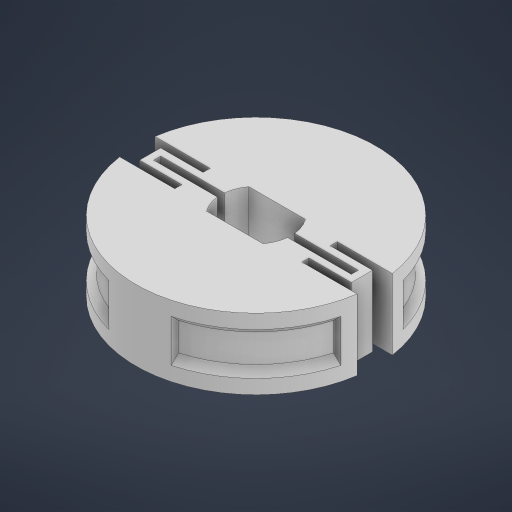
# Autodesk Inventor part: motor_grip
Saved by Autodesk Inventor 2024 (Build 280153000, 153)
## iProperties
Created: 2024-10-06
Part Number: motor_grip
Material: Generic
Document SubType Name: Modeling
Designer: loren
Density: 1 g/cm^3
Appearance: Default
Author: loren
## iProperties of the stored document shaft-grip_3DPrint.ipt
Created: 2026-02-06
Part Number: shaft-grip_3DPrint
Material: Generic
Document SubType Name: Modeling
Designer: lokies
Density: 1 g/cm^3
Appearance: Default
Author: lokies
Autodesk Inventor part; units mm, degrees
ref_plane "YZ Plane" through (0, 0, 0) normal (1, 0, 0) x (0, 1, 0)
ref_plane "XZ Plane" through (0, 0, 0) normal (0, 1, 0) x (-1, 0, 0)
ref_plane "XY Plane" through (0, 0, 0) normal (0, 0, 1) x (1, 0, 0)
sketch "Sketch1" plane through (0, 0, 0) normal (0, 0, 1) x (1, 0, 0)
  circle A0 centre (0, 0) radius 8.5
  circle A1 centre (0, 0) radius 2.5
  line L0 (-2, 1.5) -> (2, 1.5)
  line L1 (-2, -1.5) -> (2, -1.5)
  dimension "d0" = 17
  dimension "d42" = 5
  dimension "d43" = 3
  constraints: 4 end point, 4 point on circle, 2 centre point, 2 coincident, 2 horizontal, 1 parallel
  measures "d0" diameter of A0
  measures "d42" diameter of A1
  measures "d43" distance between parallel lines of L1 L0
extrude "Extrusion1" add sketch "Sketch1" along normal mid plane 5 contours A0 | L0 A1 | A1 L1
sketch "Sketch5" plane through (0, 0, 2.5) normal (0, 0, 1) x (1, 0, 0)
  line L0 (0, 0.25) -> (7, 0.25)
  line L1 (7, 0.25) -> (7, -0.25)
  line L2 (7, -0.25) -> (0, -0.25)
  line L3 (0, -0.25) -> (0, 0.25)
  circle A0 centre (0, 0) radius 8.5 projected
  line L4 (7.5, 0.75) -> (4.5, 0.75)
  line L5 (4.5, 0.75) -> (4.5, 1.25)
  line L6 (4.5, 1.25) -> (8.4076, 1.25)
  line L7 (7.5, -0.75) -> (4.5, -0.75)
  line L8 (4.5, -0.75) -> (4.5, -1.25)
  line L9 (4.5, -1.25) -> (8.4076, -1.25)
  line L10 (7.5, 0.75) -> (7.5, -0.75)
  point P0 (8.402, -1.287)
  point P1 (8.402, 1.287)
  dimension "d19" = 0.5
  dimension "d21" = 0.5
  dimension "d22" = 0.5
  dimension "d28" = 7
  dimension "d29" = 0.5
  dimension "d44" = 2.5
  dimension "d45" = 0.5
  constraints: 22 end point, 4 parallel, 3 horizontal, 3 perpendicular, 2 equal length, 2 point on circle, 1 coincident, 1 midpoint, 1 vertical
  measures "d19" distance between parallel lines of L0 L4
  measures "d21" distance between parallel lines of L4 L6
  measures "d22" distance between parallel lines of L7 L2
  measures "d28" distance from line of point (0, 0) L1
  measures "d29" distance between parallel lines of L1 L10
  measures "d44" distance between parallel lines of L1 L5
  measures "d45" distance between parallel lines of L2 L0
extrude "Extrusion5" cut sketch "Sketch5" against normal through all contours L0 L1 L2 L3 | A0 L9 L8 L7 L10 L4 L5 L6 picked at (6.8025, -1.0833)
pattern_circular "Circular Pattern2" count 2 over 360 about axis through (0, 0, -10) along (0, 0, 1) of "Extrusion5"
sketch "Sketch6" plane through (0, 0, 0) normal (0, 0, 1) x (1, 0, 0)
  arc A0 (7.6916, 2.2) -> (2.2, 7.6916) centre (0, 0) ccw
  line L0 (2.2, 7.6916) -> (2.2, 8.2104)
  arc A1 (8.4076, 1.25) -> (-8.4076, 1.25) centre (0, 0) ccw projected
  line L1 (7.6916, 2.2) -> (8.2104, 2.2)
  dimension "d30" = 60
  dimension "d31" = 0.5
  constraints: 4 end point, 4 point on circle, 1 centre point, 1 coincident, 1 horizontal, 1 perpendicular, 1 vertical
  measures "d31" radial gap between concentric circles of A1 A0
extrude "Extrusion6" cut sketch "Sketch6" along normal mid plane 3
chamfer "Chamfer2" distance 0.5 angle 45 2 edges at (5.6569, 5.6569, -1.5) (5.6569, 5.6569, 1.5)
pattern_circular "Circular Pattern3" count 4 over 360 about axis through (0, 0, -10) along (0, 0, 1) of "Extrusion6", "Chamfer2"
equation "\"d19\" = d18"
equation "\"d21\" = d19"
equation "\"d22\" = d19"
equation "\"d29\" = d19"
equation "\"d45\" = d29"
equation "\"d18\" = 0.5"
body "Solid1"
